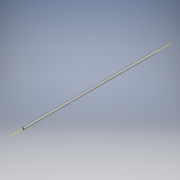
# Autodesk Inventor part: 12 Inch Hex Axle
Saved by Autodesk Inventor 2019 (Build 230136000, 136)
## iProperties
Part Number: 12 Inch Hex Axle
Material: Generic
Document SubType Name: Modeling
Designer: Delta
Appearance: Default
Author: Delta
Autodesk Inventor part; units mm, degrees
ref_plane "YZ Plane" through (0, 0, 0) normal (1, 0, 0) x (0, 1, 0)
ref_plane "XZ Plane" through (0, 0, 0) normal (0, 1, 0) x (-1, 0, 0)
ref_plane "XY Plane" through (0, 0, 0) normal (0, 0, 1) x (1, 0, 0)
sketch "Sketch1" plane through (0, 0, 0) normal (0, 0, 1) x (1, 0, 0)
  circle A0 centre (0, 0) radius 1.135
  line L0 (0, 1.135) -> (0.9829, 0.5675)
  line L1 (0, 1.135) -> (1.135, 1.135) construction
  line L2 (0.9829, 0.5675) -> (0.9829, -0.5676)
  line L3 (0.9829, -0.5676) -> (0, -1.135)
  line L4 (0, -1.135) -> (-0.9829, -0.5676)
  line L5 (-0.9829, -0.5676) -> (-0.9829, 0.5676)
  line L6 (0, 1.135) -> (-0.9829, 0.5676)
  dimension "d0" = 2.27
  dimension "d1" = 30
  dimension "d2" = 120
  dimension "d3" = 1.1351
  constraints: 14 end point, 5 point on circle, 1 centre point, 1 coincident, 1 equal length, 1 horizontal, 1 vertical
  measures "d0" diameter of A0
  measures "d1" angle of L0 L1
  measures "d2" angle of L0 L2
  measures "d3" distance of L0.end L2.end
extrude "Extrusion1" add sketch "Sketch1" along normal blind 120 contours L2 L3 L4 L5 L6 L0
fillet "Fillet1" radius 0.1 12 edges at (0.4914, 0.8513, 120) (-0.4914, 0.8513, 120) (-0.9829, 0, 120) (-0.4914, -0.8513, 120) (0.4914, -0.8513, 120) (0.9829, 0, 120) (0.4914, 0.8513, 0) (-0.4914, 0.8513, 0) (-0.9829, 0, 0) (-0.4914, -0.8513, 0) (0.4914, -0.8513, 0) (0.9829, 0, 0)
body "Solid1"
